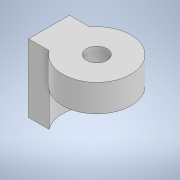
# Autodesk Inventor part: KeelHook
Saved by Autodesk Inventor 2020 (Build 240168000, 168)
## iProperties
Created: 2021-05-05
Part Number: KeelHook
Material: Generic
Document SubType Name: Modeling
Designer: chick
Density: 1 g/cm^3
Appearance: Default
Author: chick
Autodesk Inventor part; units mm, degrees
ref_plane "YZ Plane" through (0, 0, 0) normal (1, 0, 0) x (0, 1, 0)
ref_plane "XZ Plane" through (0, 0, 0) normal (0, 1, 0) x (-1, 0, 0)
ref_plane "XY Plane" through (0, 0, 0) normal (0, 0, 1) x (1, 0, 0)
sketch "Sketch1" plane through (0, 0, 0) normal (0, 1, 0) x (-1, 0, 0)
  circle A0 centre (50.2019, -50) radius 25
  point P0 (0, 0)
  dimension "d0" = 50
  dimension "d1" = 50
  constraints: 1 centre point
  measures "d0" diameter of A0
  measures "d1" vertical distance of point (0, 0) A0.centre
extrude "Extrusion1" add sketch "Sketch1" along normal blind 20
sketch "Sketch2" plane through (-50.2019, 20, -50) normal (0, 1, 0) x (1, 0, 0)
  line L0 (-35, -15) -> (-16.3886, -15)
  line L1 (-16.3886, -15) -> (-16.3886, 15)
  line L2 (-16.3886, 15) -> (-35, 15)
  line L3 (-35, 15) -> (-35, -15)
  circle A0 centre (0, 0) radius 25 projected
  circle A1 centre (0, 0) radius 25 projected
  point P0 (50.2019, -50)
  point P1 (0, 25)
  point P2 (0, -25)
  point P3 (-20, -15)
  point P4 (-20, 15)
  dimension "d4" = 15
  dimension "d5" = 15
  dimension "d6" = 35
  dimension "d7" = 50
  constraints: 8 end point, 3 perpendicular, 2 point on circle, 1 horizontal
  measures "d4" distance from line of L0 A0.centre
  measures "d5" distance from line of A0.centre L2
  measures "d6" distance from line of L3 A1.start
  measures "d7" diameter of A0
extrude "Extrusion2" add sketch "Sketch2" against normal blind 50 contours L3 L2 A0 L0
sketch "Sketch3" plane through (0, 0, 0) normal (0, -1, 0) x (1, 0, 0)
  arc A0 (-70.2019, -65) -> (-70.2019, -35) centre (-50.2019, -50) ccw projected
  arc A1 (-70.2019, -35) -> (-70.2019, -65) centre (-50.2019, -50) ccw projected
  circle A2 centre (-50.2019, -50) radius 7.5
  point P0 (0, 0)
  point P1 (-50.2019, -75)
  point P2 (-50.2019, -25)
  point P3 (-75.2019, -50)
  point P4 (-25.01, -50)
  dimension "d10" = 15
  dimension "d11" = 25
  constraints: 3 point on circle, 1 centre point, 1 coincident
  measures "d10" diameter of A2
  measures "d11" radius of A0
extrude "Extrusion3" cut sketch "Sketch3" against normal blind 30 contours A2
sketch "Sketch4" plane through (-85.2019, 20, -65) normal (-1, 0, 0) x (0, 0, 1)
  line L0 (0, -20) -> (0, -50) projected
  line L1 (30, -20) -> (30, -50) projected
  line L2 (30, -50) -> (0, -50) projected
  line L3 (40, -20) -> (-10, -20) projected
  circle A0 centre (15, -35) radius 6
  point P0 (65, -20)
  point P1 (0, -35)
  point P2 (30, -35)
  point P3 (15, -50)
  point P4 (15, -20)
  point P5 (15, -20)
  dimension "d14" = 30
  dimension "d15" = 15
  dimension "d16" = 15
  dimension "d17" = 12
  constraints: 4 midpoint, 1 centre point, 1 coincident
  measures "d14" distance from line of L0 point (30, -35)
  measures "d15" distance of point (30, -35) A0.centre
  measures "d16" distance of A0.centre point (0, -35)
  measures "d17" diameter of A0
extrude "Extrusion4" cut sketch "Sketch4" against normal blind 30 contours A0
equation "\"d10\" = 0.6 * d11"
equation "\"d15\" = 0.5 * d14"
equation "\"d16\" = 0.5 * d14"
equation "\"d17\" = 0.4 * d14"
body "Solid1"
